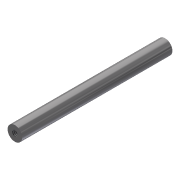
# Autodesk Inventor part: Axle Nick
Saved by Autodesk Inventor 2015 (Build 190159000, 159)
## iProperties
Created: 2014-01-20
Part Number: Axle Nick
Material: Stainless Steel
Document SubType Name: Modeling
Designer: Nick
Density: 8 g/cm^3
Appearance: Semi-Polished
Mass: 125.271 g
Surface Area: 63.0385 cm^2
Volume: 15.6589 cm^3
Author: Nick
Autodesk Inventor part; units mm, degrees
ref_plane "YZ Plane" through (0, 0, 0) normal (1, 0, 0) x (0, 1, 0)
ref_plane "XZ Plane" through (0, 0, 0) normal (0, 1, 0) x (-1, 0, 0)
ref_plane "XY Plane" through (0, 0, 0) normal (0, 0, 1) x (1, 0, 0)
sketch "Sketch1" plane through (0, 0, 0) normal (0, 0, 1) x (1, 0, 0)
  circle A0 centre (0, 0) radius 6.35
  dimension "d0" = 12.7
  constraints: 1 centre point, 1 coincident
  measures "d0" diameter of A0
extrude "Extrusion1" add sketch "Sketch1" along normal blind 131.572
sketch "Sketch2" plane through (0, 0, 131.572) normal (0, 0, 1) x (1, 0, 0)
  circle A0 centre (0, 0) radius 6.35 projected
  constraints: 1 coincident
hole "Hole1" at (0, 0, 131.572) direction (0, 0, -1) diameter 4.9784 depth 25.4 tip angle 118 thread size "1/4-20 UNC" class "2B" standard "ANSI Unified Screw Threads"
sketch "Sketch3" plane through (0, 0, 0) normal (0, 0, -1) x (-1, 0, 0)
  circle A0 centre (0, 0) radius 6.35 projected
  constraints: 1 coincident
hole "Hole2" at (0, 0, 0) direction (0, 0, 1) diameter 4.9784 depth 25.4 tip angle 118 thread size "1/4-20 UNC" class "2B" standard "ANSI Unified Screw Threads"
body "Solid1"
